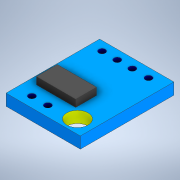
# Autodesk Inventor part: tof
Saved by Autodesk Inventor 2022 (Build 260153000, 153)
## iProperties
Created: 2022-12-09
Part Number: tof
Material: Generic
Document SubType Name: Modeling
Designer: Kamil
Density: 1 g/cm^3
Appearance: Default
Author: Kamil
Autodesk Inventor part; units mm, degrees
ref_plane "YZ Plane" through (0, 0, 0) normal (1, 0, 0) x (0, 1, 0)
ref_plane "XZ Plane" through (0, 0, 0) normal (0, 1, 0) x (-1, 0, 0)
ref_plane "XY Plane" through (0, 0, 0) normal (0, 0, 1) x (1, 0, 0)
sketch "Sketch1" plane through (0, 0, 0) normal (0, 1, 0) x (-1, 0, 0)
  line L0 (14.7075, 31.6187) -> (4.3075, 31.6187)
  line L1 (4.3075, 31.6187) -> (4.3075, 44.7187)
  line L2 (4.3075, 44.7187) -> (14.7075, 44.7187)
  line L3 (14.7075, 44.7187) -> (14.7075, 31.6187)
  line L4 (13.5937, 38.6629) -> (8.0964, 38.6629)
  line L5 (8.0964, 38.6629) -> (8.0964, 41.5823)
  line L6 (8.0964, 41.5823) -> (13.5937, 41.5823)
  line L7 (13.5937, 41.5823) -> (13.5937, 38.6629)
  circle A0 centre (6.5746, 42.8557) radius 1.4817
  point P0 (0, 0)
  dimension "d0" = 10.4
  dimension "d1" = 13.1
  constraints: 16 end point, 4 parallel, 2 horizontal, 2 perpendicular, 1 centre point
  measures "d0" distance of L1.end L2.end
  measures "d1" distance of L0.end L1.end
extrude "Extrusion1" add sketch "Sketch1" along normal blind 2
extrude "Extrusion2" add sketch "Sketch1" along normal blind 3 contours L4 L5 L6 L7
sketch "Sketch2" plane through (0, 2, 0) normal (0, 1, 0) x (1, 0, 0)
  line L0 (-13.674, -32.9177) -> (-5.5891, -32.9177)
  line L1 (-13.5937, -43.2778) -> (-9.2456, -43.2778)
  point P0 (0, 0)
  point P1 (-13.0646, -32.9177)
  point P2 (-6.5641, -32.9177)
  point P3 (-10.952, -32.9177)
  point P4 (-8.8393, -32.9177)
  point P5 (-12.5364, -43.2778)
  point P6 (-10.3019, -43.2778)
  constraints: 6 point on line, 4 end point, 2 horizontal
hole "Hole1" at (-13.0646, 2, 32.9177) at (-6.5641, 2, 32.9177) at (-10.952, 2, 32.9177) at (-8.8393, 2, 32.9177) at (-12.5364, 2, 43.2778) at (-10.3019, 2, 43.2778) direction (0, -1, 0) diameter 0.9 end through all
sketch "Sketch3" plane through (0, 0, 0) normal (0, -1, 0) x (1, 0, 0)
  circle A0 centre (-12.5364, 43.2778) radius 0.45 projected
  circle A1 centre (-10.952, 32.9177) radius 0.45 projected
  circle A2 centre (-13.0646, 32.9177) radius 0.45 projected
  circle A3 centre (-6.5641, 32.9177) radius 0.45 projected
  circle A4 centre (-8.8393, 32.9177) radius 0.45 projected
  circle A5 centre (-10.3019, 43.2778) radius 0.45 projected
  line L0 (-14.7075, 44.7187) -> (-4.3075, 44.7187) projected
  line L1 (-14.7075, 31.6187) -> (-14.7075, 44.7187) projected
  line L2 (-4.3075, 31.6187) -> (-14.7075, 31.6187) projected
  line L3 (-4.3075, 44.7187) -> (-4.3075, 31.6187) projected
  circle A6 centre (-6.5746, 42.8557) radius 1.4817 projected
  point P0 (0, 0)
extrude "Extrusion3" cut sketch "Sketch3" against normal blind 0.4
body "Solid1"
